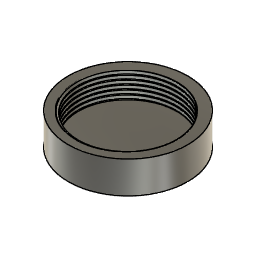
StampOutCase v1 (Autodesk Fusion 360 design; units mm, degrees)
Autodesk Fusion 360 part; units mm, degrees
sketch "Sketch1" plane through (0, 0, 0) normal (0, 0, 1) x (1, 0, 0)
  circle A0 centre (0, 0) radius 28
  dimension "d1" = 56
  constraint coincident A0.centre origin
  measures "d1" diameter of A0
extrude "Extrude1" add sketch "Sketch1" along normal blind 15
hole "Hole1" at (0, 0, 15) direction (0, 0, -1) diameter 30 depth 12 tip angle 180
thread "Thread1" "ISO Metric profile 48.0 M48x2 6H" major diameter 48.2625 minor diameter 46.0225 pitch 2 angle 60 modelled right hand crest width 0.5401 on face at (0.7477, -14.9814, 11) crest through (23.0113, 0, 14.5)
